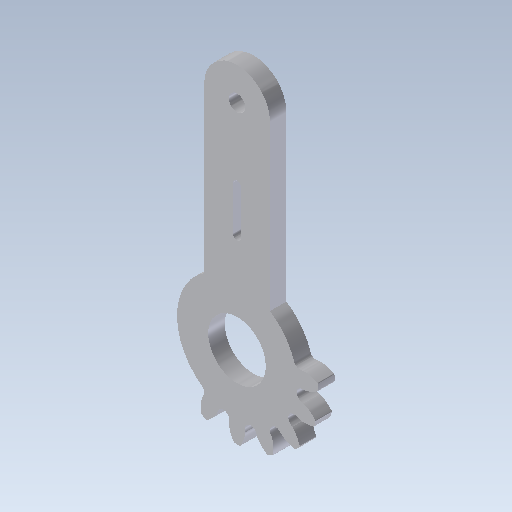
# Autodesk Inventor part: gear2
Saved by Autodesk Inventor 2020.3 (Build 243373000, 373)
## iProperties
Created: 2016-01-08
Part Number: gear2
Material: ABS Plastic
Document SubType Name: Modeling
Designer: Nanjar
Density: 1.06 g/cm^3
Appearance: Cool White
Author: Nanjar
Autodesk Inventor part; units mm, degrees
ref_plane "YZ Plane" through (0, 0, 0) normal (1, 0, 0) x (0, 1, 0)
ref_plane "XZ Plane" through (0, 0, 0) normal (0, 1, 0) x (-1, 0, 0)
ref_plane "XY Plane" through (0, 0, 0) normal (0, 0, 1) x (1, 0, 0)
sketch "Sketch1" plane through (0, 0, 0) normal (0, 0, 1) x (1, 0, 0)
  spline S0 degree 3 poles (-2.528711, 14.658487) (-2.448915, 14.573394) (-2.289324, 14.403208) (-2.065031, 14.134402) (-1.853138, 13.855809) (-1.656553, 13.566132) (-1.477372, 13.265364) (-1.345502, 13.005004) (-1.253074, 12.790735) (-1.19212, 12.626748) (-1.138717, 12.45985) (-1.117351, 12.345121) (-1.10667, 12.287772) knots 0 0 0 0 0.12500929 0.25001935 0.37502787 0.50003343 0.62503428 0.75002663 0.81253235 0.87503596 0.93753456 1 1 1 1
  spline S1 degree 3 poles (-1.10667, 12.287772) (-1.101319, 12.20544) (-1.093291, 12.081931) (-1.068438, 11.918715) (-1.041149, 11.797985) (-1.007909, 11.678696) (-0.963749, 11.562999) (-0.912304, 11.450327) (-0.848677, 11.343926) (-0.774286, 11.244774) (-0.688272, 11.155399) (-0.59113, 11.078214) (-0.484037, 11.015401) (-0.368658, 10.969626) (-0.247524, 10.941846) (-0.123639, 10.935736) (0, 10.938383) (0.123639, 10.935736) (0.247524, 10.941846) (0.368658, 10.969626) (0.484037, 11.015401) (0.59113, 11.078214) (0.688272, 11.155399) (0.774286, 11.244774) (0.848677, 11.343926) (0.912304, 11.450327) (0.963749, 11.562999) (1.007909, 11.678696) (1.041149, 11.797985) (1.068438, 11.918715) (1.093291, 12.081931) (1.101319, 12.20544) (1.10667, 12.287772) knots 0 0 0 0 0.06249765 0.09375418 0.12500812 0.15626686 0.18751701 0.21877048 0.25002912 0.28128175 0.31252886 0.34377646 0.37503042 0.40627698 0.4375148 0.46874353 0.5 0.53125647 0.5624852 0.59372302 0.62496958 0.65622354 0.68747114 0.71871825 0.74997088 0.78122952 0.81248299 0.84373314 0.87499188 0.90624582 0.93750235 1 1 1 1
  spline S2 degree 3 poles (1.10667, 12.287772) (1.117351, 12.345121) (1.138717, 12.45985) (1.19212, 12.626748) (1.253074, 12.790735) (1.345502, 13.005004) (1.477372, 13.265364) (1.656553, 13.566132) (1.853138, 13.855809) (2.065031, 14.134402) (2.289324, 14.403208) (2.448915, 14.573394) (2.528711, 14.658487) knots 0 0 0 0 0.06246544 0.12496404 0.18746765 0.24997337 0.37496572 0.49996657 0.62497213 0.74998065 0.87499071 1 1 1 1
  circle A0 centre (0, 0) radius 10.9375 construction
  circle A1 centre (0, 0) radius 12.333466 construction
  circle A2 centre (0, 0) radius 13.125 construction
  circle A3 centre (0, 0) radius 14.875
  point P0 (-2.29184, 14.400954)
  point P1 (-2.067096, 14.13277)
  point P2 (-1.855687, 13.853959)
  point P3 (-1.65945, 13.564278)
  point P4 (-1.480858, 13.263413)
  point P5 (-1.32349, 12.95095)
  point P6 (-1.254468, 12.790187)
  point P7 (-1.193375, 12.626253)
  point P8 (-1.142267, 12.458951)
  point P9 (-1.085901, 12.041264)
  point P10 (-1.066996, 11.918995)
  point P11 (-1.040159, 11.79823)
  point P12 (-1.006086, 11.679284)
  point P13 (-0.962537, 11.563507)
  point P14 (-0.910277, 11.451379)
  point P15 (-0.846878, 11.345126)
  point P16 (-0.772343, 11.246396)
  point P17 (-0.686418, 11.157431)
  point P18 (-0.589478, 11.080614)
  point P19 (-0.482645, 11.018235)
  point P20 (-0.367682, 10.97262)
  point P21 (-0.247056, 10.945455)
  point P22 (-0.123721, 10.937196)
  point P23 (0, 10.9375)
  point P24 (0.123721, 10.937196)
  point P25 (0.247056, 10.945455)
  point P26 (0.367682, 10.97262)
  point P27 (0.482645, 11.018235)
  point P28 (0.589478, 11.080614)
  point P29 (0.686418, 11.157431)
  point P30 (0.772343, 11.246396)
  point P31 (0.846878, 11.345126)
  point P32 (0.910277, 11.451379)
  point P33 (0.962537, 11.563507)
  point P34 (1.006086, 11.679284)
  point P35 (1.040159, 11.79823)
  point P36 (1.066996, 11.918995)
  point P37 (1.085901, 12.041264)
  point P38 (1.142267, 12.458951)
  point P39 (1.193375, 12.626253)
  point P40 (1.254468, 12.790187)
  point P41 (1.32349, 12.95095)
  point P42 (1.480858, 13.263413)
  point P43 (1.65945, 13.564278)
  point P44 (1.855687, 13.853959)
  point P45 (2.067096, 14.13277)
  point P46 (2.29184, 14.400954)
  constraints: 4 centre point, 2 point on circle, 109 other
extrude "Extrusion1" add sketch "Sketch1" against normal blind 3
extrude "Extrusion2" cut sketch "Sketch1" against normal through all contours A3 S2 S1 S0 picked at (0.259388, 13.581093)
fillet "Fillet1" radius 0.2 2 edges at (-2.5287, 14.6585, -1.5) (2.5287, 14.6585, -1.5)
pattern_circular "Circular Pattern1" count 15 over 360 about axis through (0, 0, 0) along (0, 0, -1) of "Fillet1", "Extrusion2"
sketch "Sketch9" plane through (0, 0, 0) normal (0, 1, 0) x (-1, 0, 0)
  line L0 (-6, -3) -> (6, -3)
  line L1 (6, -3) -> (6, 0)
  line L2 (6, 0) -> (-6, 0)
  line L3 (-6, 0) -> (-6, -3)
  line L4 (-6, -3) -> (6, 0) construction
  line L5 (6, -3) -> (-6, 0) construction
  line L6 (0, 0) -> (0, -1.5) construction
  point P0 (0, 0)
  dimension "d38" = 3
  dimension "d70" = 12
  constraints: 14 end point, 2 midpoint, 2 parallel, 1 coincident, 1 horizontal, 1 perpendicular
  measures "d38" distance of L1.end L0.end
  measures "d70" distance of L0.start L0.end
extrude "Extrusion8" add sketch "Sketch9" along normal blind 45
sketch "Sketch10" plane through (0, 0, 0) normal (0, 0, 1) x (1, 0, 0)
  circle A0 centre (0, 0) radius 5.25
  dimension "d41" = 10.5
  constraints: 1 centre point, 1 coincident
  measures "d41" diameter of A0
extrude "Extrusion9" cut sketch "Sketch10" against normal through all
fillet "Fillet8" radius 6 2 edges at (6, 45, -1.5) (-6, 45, -1.5)
sketch "Sketch15" plane through (0, 0, 0) normal (0, 0, 1) x (1, 0, 0)
  arc A0 (0.75, 26) -> (-0.75, 26) centre (0, 26) ccw
  arc A1 (-0.75, 18) -> (0.75, 18) centre (0, 18) ccw
  line L0 (0.75, 18) -> (0.75, 26)
  line L1 (-0.75, 18) -> (-0.75, 26)
  line L2 (0, 18) -> (0, 26) construction
  line L3 (0, 26) -> (-0.75, 26) construction
  point P0 (0, 0)
  dimension "d62" = 1.5
  dimension "d68" = 18
  dimension "d69" = 8
  constraints: 8 end point, 4 point on circle, 2 centre point, 2 vertical, 1 horizontal, 1 parallel
  measures "d62" diameter of A0
  measures "d68" distance of point (0, 0) L2.start
  measures "d69" distance of L2.start L2.end
extrude "Extrusion14" cut sketch "Sketch15" against normal through all
sketch "Sketch16" plane through (0, 0, 0) normal (0, 0, 1) x (1, 0, 0)
  arc A0 (10.401991, 3.379812) -> (6, 9.144646) centre (0, 0) ccw
  line L0 (10.380603, 3.444941) -> (10.42297, 3.31455) construction
  line L1 (10.401991, 3.379812) -> (18.259665, 5.932925)
  line L2 (18.259665, 5.932925) -> (6, 14.430056)
  line L3 (6, 14.430056) -> (6, 9.144646)
  constraints: 8 end point, 3 point on circle, 1 centre point, 1 coincident, 1 perpendicular, 4 other
extrude "Extrusion15" cut sketch "Sketch16" against normal through all
sketch "Sketch17" plane through (0, 0, 0) normal (0, 0, 1) x (1, 0, 0)
  arc A0 (-6, 9.144646) -> (-6.484116, -8.807995) centre (0, 0) ccw
  line L0 (-6.484116, -8.807995) -> (-9.404184, -12.774603)
  line L1 (-15.158525, -5.054184) -> (-16.217524, -0.687437)
  line L2 (-15.158525, 5.742128) -> (-11.676881, 12.056297)
  line L3 (-6, 10.758418) -> (-6, 39)
  line L4 (-6, 13.433022) -> (-11.676881, 12.056297)
  line L5 (-15.158525, 5.742128) -> (-16.217524, -0.687437)
  line L6 (-15.158525, -5.054184) -> (-9.404184, -12.774603)
  line L7 (-6, 13.433022) -> (-6, 9.144646)
  constraints: 14 end point, 2 coincident, 2 point on circle, 1 centre point, 1 collinear, 1 perpendicular, 1 point on line, 4 other
extrude "Extrusion16" cut sketch "Sketch17" against normal through all
sketch "Sketch18" plane through (0, 0, 0) normal (0, 0, 1) x (1, 0, 0)
  arc A0 (6, 39) -> (-6, 39) centre (0, 39) ccw projected
  circle A1 centre (0, 39) radius 1.5
  point P0 (0, 0)
  dimension "d75" = 3
  constraints: 1 centre point, 1 coincident
  measures "d75" diameter of A1
extrude "Extrusion17" cut sketch "Sketch18" against normal through all
equation "\"d0\" = FaceWidth"
equation "\"Module\" = 1.75"
equation "\"PressureAngle\" = 20deg"
equation "\"UnitProfileClearance\" = 0.25"
equation "\"UnitRoundRadius\" = 0.35"
equation "\"HeadDiameter\" = 29.75"
equation "\"RootDiameter\" = 21.875"
equation "\"BaseDiameter\" = 24.66693"
equation "\"PitchDiameter\" = 26.25"
equation "\"FaceWidth\" = 3"
equation "\"HelixAngle\" = 0"
equation "\"UnitCorrection\" = 0"
equation "\"UnitAddendumModification\" = 0"
equation "\"CircularPitch\" = 5.497787"
equation "\"UnitBacklashShift\" = 0"
equation "\"TotalToolShift\" = 0"
equation "\"IsInternal\" = 0"
body "Solid1"
